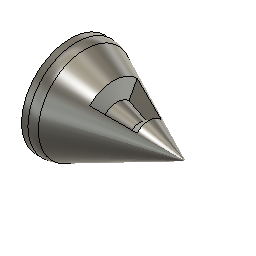
Aguja Bolsillo Radial v0 (Autodesk Fusion 360 design; units mm, degrees)
Autodesk Fusion 360 part; units mm, degrees
sketch "Sketch1" plane through (0, 0, 0) normal (0, 1, 0) x (1, 0, 0)
  line L0 (0, 0) -> (272, 0)
  line L1 (0, 0) -> (0, -115)
  line L2 (0, -115) -> (14.7579, -115)
  line L3 (35.0449, -110.5022) -> (272, 0)
  arc A0 (14.7579, -115) -> (35.0449, -110.5022) centre (14.7579, -67) ccw
  point P0 (25.4, -115)
  dimension "d1" = 272
  dimension "d2" = 115
  dimension "d3" = 25.4
  dimension "d4" = 48
  constraint coincident L0.start L1.start
  constraint horizontal L0
  constraint perpendicular L0 L1
  constraint perpendicular L1 L2
  constraint coincident P0 L2
  constraint coincident P0 L3
  constraint tangent L2 A0
  constraint tangent L3 A0
  measures "d1" distance of L0.start L0.end
  measures "d2" distance of L0.start L1.end
  measures "d3" distance of L1.end P0
  measures "d4" radius of A0
revolve "Revolve1" add sketch "Sketch1" angle 360 about axis through (0, 0, 0) along (1, 0, 0)
ref_plane "WorkPlane1" through (0, 0, 0) normal (0, 0, 1) x (1, 0, 0)
sketch "Sketch2" plane through (0, 0, 0) normal (0, 0, 1) x (1, 0, 0)
  line L0 (100.5395, 84.3629) -> (110, 40)
  line L1 (110, 40) -> (163.6315, 25.2684)
  line L2 (163.6315, 25.2684) -> (189.7167, 43.1547)
  line L3 (189.7167, 43.1547) -> (100.5395, 84.3629)
revolve "Revolve2" cut sketch "Sketch2" angle 45 about axis through (1.75, 0, 0) along (1, 0, 0) second angle 45
